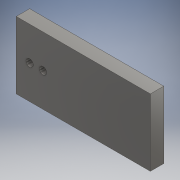
# Autodesk Inventor part: MotorFixer
Saved by Autodesk Inventor 2017 (Build 210142000, 142)
## iProperties
Created: 2016-12-12
Part Number: MotorFixer
Material: Steel, Carbon
Document SubType Name: Modeling
Designer: umr
Density: 7.85 g/cm^3
Appearance: Semi-Polished
Mass: 465.405 g
Surface Area: 157.758 cm^2
Volume: 59.2873 cm^3
Author: umr
Autodesk Inventor part; units mm, degrees
ref_plane "YZ Plane" through (0, 0, 0) normal (1, 0, 0) x (0, 1, 0)
ref_plane "XZ Plane" through (0, 0, 0) normal (0, 1, 0) x (-1, 0, 0)
ref_plane "XY Plane" through (0, 0, 0) normal (0, 0, 1) x (1, 0, 0)
sketch "Sketch1" plane through (0, 0, 0) normal (0, 1, 0) x (-1, 0, 0)
  line L0 (0, 0) -> (100, 0)
  line L1 (100, 0) -> (100, -50)
  line L2 (100, -50) -> (0, -50)
  line L3 (0, -50) -> (0, 0)
  dimension "d0" = 100
  dimension "d1" = 50
  constraints: 8 end point, 2 parallel, 1 horizontal, 1 perpendicular
  measures "d0" distance of L1.end L2.end
  measures "d1" distance of L0.end L1.end
extrude "Extrusion1" add sketch "Sketch1" along normal blind 10
sketch "Sketch2" plane through (0, 10, 0) normal (0, 1, 0) x (1, 0, 0)
  line L0 (-100, 50) -> (-100, 0) projected
  line L1 (-100, 0) -> (0, 0) projected
  circle A0 centre (-90, 25) radius 2.75
  circle A1 centre (-80, 25) radius 2.75
  dimension "d4" = 5.5
  dimension "d5" = 25
  dimension "d6" = 10
  dimension "d9" = 10
  dimension "d32" = 50
  constraints: 2 centre point, 1 horizontal, 2 other
  measures "d4" diameter of A0
  measures "d5" distance from line of L1 A0.centre
  measures "d6" distance from line of L0 A0.centre
  measures "d9" distance of A0.centre A1.centre
  measures "d32" distance of L0.start L0.end
extrude "Extrusion4" cut sketch "Sketch2" against normal blind 10
equation "\"d5\" = 0.5 * d32"
body "Solid1"
